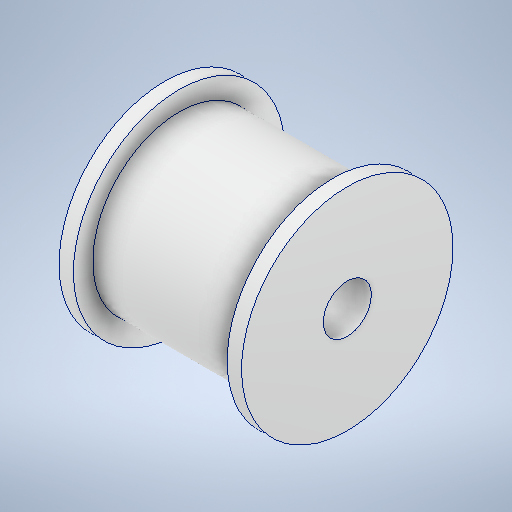
# Autodesk Inventor part: Belt_Bearing
Saved by Autodesk Inventor 2025.1 (Build 291241020, 241B)
## iProperties
Created: 2024-11-07
Part Number: Belt_Bearing
Material: Aluminum 6061
Document SubType Name: Modeling
Designer: leon-
Density: 2.7 g/cm^3
Appearance: Aluminum - Flat
Author: leon-
Autodesk Inventor part; units mm, degrees
ref_plane "YZ Plane" through (0, 0, 0) normal (1, 0, 0) x (0, 1, 0)
ref_plane "XZ Plane" through (0, 0, 0) normal (0, 1, 0) x (-1, 0, 0)
ref_plane "XY Plane" through (0, 0, 0) normal (0, 0, 1) x (1, 0, 0)
sketch "Sketch1" plane through (0, 0, 0) normal (0, 0, 1) x (1, 0, 0)
  line L0 (9.5, 2.5) -> (9.5, 11)
  line L1 (9.5, 11) -> (8, 11)
  line L2 (8, 11) -> (8, 8.98)
  line L3 (8, 8.98) -> (0, 8.98)
  line L4 (9.5, 2.5) -> (0, 2.5)
  line L5 (0, 2.5) -> (0, 8.98)
  line L6 (-1.9, 0) -> (11.4, 0) projected
  line L7 (0, 0.8) -> (0, 12.7) projected
  point P0 (0, 5.74)
  dimension "d0" = 9.5
  dimension "d1" = 8
  dimension "d2" = 8.98
  dimension "d3" = 11
  dimension "d4" = 2.5
  constraints: 12 end point, 4 perpendicular, 1 collinear, 1 horizontal, 1 midpoint, 1 vertical
  measures "d0" distance between parallel lines of L5 L0
  measures "d1" distance from line of point (0, 5.74) L2
  measures "d2" distance between parallel lines of L6 L3
  measures "d3" distance between parallel lines of L6 L1
  measures "d4" distance between parallel lines of L6 L4
revolve "Revolution1" add sketch "Sketch1" angle 360 about axis through (-10, 0, 0) along (1, 0, 0)
mirror "Mirror1" about plane through (0, 0, 0) normal (1, 0, 0) of "Revolution1"
body "Solid1"
